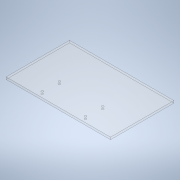
# Autodesk Inventor part: Top-Lid
Saved by Autodesk Inventor 2022 (Build 260153000, 153)
## iProperties
Company: El Camino College
Created: 2022-12-16
Part Number: Top-Lid
Material: Polycarbonate, Clear
Document SubType Name: Modeling
Designer: Edgar Tejada
Density: 1.2 g/cm^3
Appearance: Polycarbonate - Clear
Project: Parametric-Modeling
Author: Edgar Tejada
Title: Battery Pack Top-Lid
Autodesk Inventor part; units mm, degrees
ref_plane "YZ Plane" through (0, 0, 0) normal (1, 0, 0) x (0, 1, 0)
ref_plane "XZ Plane" through (0, 0, 0) normal (0, 1, 0) x (-1, 0, 0)
ref_plane "XY Plane" through (0, 0, 0) normal (0, 0, 1) x (1, 0, 0)
sketch "Sketch1" plane through (0, 0, 0) normal (0, 1, 0) x (-1, 0, 0)
  line L0 (70, -42.5) -> (-70, -42.5)
  line L1 (-70, -42.5) -> (-70, 42.5)
  line L2 (-70, 42.5) -> (70, 42.5)
  line L3 (70, 42.5) -> (70, -42.5)
  line L4 (70, -42.5) -> (-70, 42.5) construction
  line L5 (-70, -42.5) -> (70, 42.5) construction
  point P0 (0, 0)
  point P1 (0, 0)
  point P2 (0, 0)
  dimension "d0" = 140
  dimension "d1" = 85
  constraints: 12 end point, 3 midpoint, 2 parallel, 1 coincident, 1 horizontal, 1 perpendicular
  measures "d0" distance of L1.end L2.end
  measures "d1" distance of L2.end L0.start
extrude "Lid" add sketch "Sketch1" against normal blind 3
sketch "Sketch2" plane through (0, 0, 0) normal (0, 1, 0) x (-1, 0, 0)
  line L0 (29, 12) -> (-29, 12) construction
  line L1 (-29, 12) -> (-29, 35) construction
  line L2 (-29, 35) -> (29, 35) construction
  line L3 (29, 35) -> (29, 12) construction
  line L4 (29, 12) -> (-29, 35) construction
  line L5 (-29, 12) -> (29, 35) construction
  circle A0 centre (29, 12) radius 1.4
  circle A1 centre (-29, 12) radius 1.4
  circle A2 centre (-29, 35) radius 1.4
  circle A3 centre (29, 35) radius 1.4
  point P0 (0, 0)
  point P1 (0, 0)
  point P2 (0, 23.5)
  point P3 (0, 23.5)
  point P4 (0, 23.5)
  dimension "d4" = 23
  dimension "d5" = 58
  dimension "d6" = 12
  dimension "d7" = 2.8
  constraints: 12 end point, 5 coincident, 4 centre point, 4 midpoint, 3 equal radius, 2 parallel, 2 vertical alignment, 1 horizontal, 1 perpendicular
  measures "d4" distance of L0.end L1.end
  measures "d5" distance of L1.end L2.end
  measures "d6" distance from line of L0 point (0, 0)
  measures "d7" diameter of A0
extrude "M3_Mount_Holes" cut sketch "Sketch2" along normal through all both and the other way through all
equation "\"d1\" = 0.607143 * d0"
equation "\"d2\" = 0.0214286 * d0"
equation "\"d4\" = 0.164286 * d0"
equation "\"d5\" = 0.414286 * d0"
equation "\"d6\" = 0.0857143 * d0"
equation "\"d7\" = 0.02 * d0"
body "Solid1"
